Autodesk Fusion 360 part; units mm, degrees
(part 4 of 5)
  spline S1159 degree 3 poles (4.1337, -1.152) (3.9623, -1.0527) (3.8179, -1.0076) (3.8179, -1.0527) knots 0 0 0 0 1 1 1 1
  spline S1160 degree 3 poles (3.8179, -1.0527) (3.8179, -1.2062) (4.224, -1.5762) (4.3323, -1.5311) knots 0 0 0 0 1 1 1 1
  spline S1161 degree 3 poles (23.384, -1.3506) (23.5284, -1.2964) (24.1241, -0.5203) (24.1241, -0.3939) knots 0 0 0 0 1 1 1 1
  spline S1162 degree 3 poles (24.1241, -0.3939) (24.1241, -0.3398) (23.9797, -0.43) (23.8082, -0.6015) knots 0 0 0 0 1 1 1 1
  spline S1163 degree 3 poles (23.8082, -0.6015) (23.4562, -0.9444) (23.4021, -0.8813) (23.6728, -0.4481) knots 0 0 0 0 1 1 1 1
  spline S1164 degree 3 poles (23.6728, -0.4481) (23.9075, -0.06) (23.7721, -0.069) (23.5284, -0.4571) knots 0 0 0 0 1 1 1 1
  spline S1165 degree 3 poles (23.5284, -0.4571) (23.384, -0.6827) (23.1584, -1.4408) (23.2487, -1.4047) knots 0 0 0 0 1 1 1 1
  spline S1166 degree 3 poles (23.2487, -1.4047) (23.2577, -1.4047) (23.3209, -1.3776) (23.384, -1.3506) knots 0 0 0 0 1 1 1 1
  spline S1167 degree 3 poles (7.2203, -1.3506) (7.4188, -1.2784) (7.3557, -0.9625) (7.1571, -0.9625) knots 0 0 0 0 1 1 1 1
  spline S1168 degree 3 poles (7.1571, -0.9625) (7.0398, -0.9625) (6.9766, -1.0257) (6.9766, -1.134) knots 0 0 0 0 1 1 1 1
  spline S1169 degree 3 poles (6.9766, -1.134) (6.9766, -1.3325) (7.0578, -1.4047) (7.2203, -1.3506) knots 0 0 0 0 1 1 1 1
  spline S1170 degree 3 poles (22.4725, -1.1159) (22.8425, -0.9174) (23.4653, -0.2766) (23.1855, -0.3849) knots 0 0 0 0 1 1 1 1
  spline S1171 degree 3 poles (23.1855, -0.3849) (23.1043, -0.412) (23.0411, -0.3939) (23.0411, -0.3398) knots 0 0 0 0 1 1 1 1
  spline S1172 degree 3 poles (23.0411, -0.3398) (23.0411, -0.2856) (22.996, -0.2405) (22.9508, -0.2405) knots 0 0 0 0 1 1 1 1
  spline S1173 degree 3 poles (22.9508, -0.2405) (22.8967, -0.2405) (22.8696, -0.2676) (22.8786, -0.3127) knots 0 0 0 0 1 1 1 1
  spline S1174 degree 3 poles (22.8786, -0.3127) (22.8877, -0.3488) (22.8245, -0.5022) (22.7433, -0.6647) knots 0 0 0 0 1 1 1 1
  spline S1175 degree 3 poles (22.7433, -0.6647) (22.5898, -0.9535) (22.3462, -1.0888) (21.9852, -1.0979) knots 0 0 0 0 1 1 1 1
  spline S1176 degree 3 poles (21.9852, -1.0979) (21.8678, -1.0979) (21.7686, -1.143) (21.7595, -1.1881) knots 0 0 0 0 1 1 1 1
  spline S1177 degree 3 poles (21.7595, -1.1881) (21.7144, -1.3596) (22.0935, -1.3235) (22.4725, -1.1159) knots 0 0 0 0 1 1 1 1
  spline S1178 degree 3 poles (-3.6278, -1.2332) (-3.6007, -1.1881) (-3.6187, -1.143) (-3.6639, -1.143) knots 0 0 0 0 1 1 1 1
  spline S1179 degree 3 poles (-3.6639, -1.143) (-3.718, -1.143) (-3.7631, -1.1881) (-3.7631, -1.2332) knots 0 0 0 0 1 1 1 1
  spline S1180 degree 3 poles (-3.7631, -1.2332) (-3.7631, -1.2874) (-3.7451, -1.3235) (-3.727, -1.3235) knots 0 0 0 0 1 1 1 1
  spline S1181 degree 3 poles (-3.727, -1.3235) (-3.7, -1.3235) (-3.6548, -1.2874) (-3.6278, -1.2332) knots 0 0 0 0 1 1 1 1
  spline S1182 degree 3 poles (5.5326, -1.152) (5.5326, -1.0979) (5.307, -0.9083) (5.0362, -0.7278) knots 0 0 0 0 1 1 1 1
  spline S1183 degree 3 poles (5.0362, -0.7278) (4.6843, -0.4932) (4.5399, -0.3398) (4.5399, -0.1954) knots 0 0 0 0 1 1 1 1
  spline S1184 degree 3 poles (4.5399, -0.1954) (4.5399, -0.0871) (4.4406, 0.1476) (4.3233, 0.3281) knots 0 0 0 0 1 1 1 1
  spline S1185 degree 3 poles (4.3233, 0.3281) (4.1518, 0.5808) (4.1067, 0.7252) (4.1518, 0.9779) knots 0 0 0 0 1 1 1 1
  spline S1186 degree 3 poles (4.1518, 0.9779) (4.1879, 1.1945) (4.1698, 1.2938) (4.0886, 1.2938) knots 0 0 0 0 1 1 1 1
  spline S1187 degree 3 poles (4.0886, 1.2938) (4.0074, 1.2938) (3.9893, 1.393) (4.0254, 1.6277) knots 0 0 0 0 1 1 1 1
  spline S1188 degree 3 poles (4.0254, 1.6277) (4.0706, 1.9345) (4.0706, 1.9526) (3.9532, 1.8082) knots 0 0 0 0 1 1 1 1
  spline S1189 degree 3 poles (3.9532, 1.8082) (3.8359, 1.6457) (3.8269, 1.6548) (3.7998, 1.8533) knots 0 0 0 0 1 1 1 1
  spline S1190 degree 3 poles (3.7998, 1.8533) (3.7818, 1.9706) (3.8179, 2.2414) (3.881, 2.458) knots 0 0 0 0 1 1 1 1
  spline S1191 degree 3 poles (3.881, 2.458) (3.9713, 2.8009) (3.9713, 2.837) (3.863, 2.7287) knots 0 0 0 0 1 1 1 1
  spline S1192 degree 3 poles (3.863, 2.7287) (3.7908, 2.6565) (3.6735, 2.476) (3.5922, 2.3316) knots 0 0 0 0 1 1 1 1
  line L74 (3.5922, 2.3316) -> (3.4388, 2.0609)
  line L75 (3.4388, 2.0609) -> (3.4839, 2.3768)
  spline S1193 degree 3 poles (3.4839, 2.3768) (3.52, 2.6475) (3.502, 2.7017) (3.3666, 2.7107) knots 0 0 0 0 1 1 1 1
  spline S1194 degree 3 poles (3.3666, 2.7107) (3.2673, 2.7197) (3.1681, 2.6475) (3.141, 2.5482) knots 0 0 0 0 1 1 1 1
  spline S1195 degree 3 poles (3.141, 2.5482) (3.0688, 2.3316) (3.2764, 1.7721) (3.3666, 1.9255) knots 0 0 0 0 1 1 1 1
  spline S1196 degree 3 poles (3.3666, 1.9255) (3.3937, 1.9706) (3.4298, 1.7811) (3.4388, 1.5013) knots 0 0 0 0 1 1 1 1
  spline S1197 degree 3 poles (3.4388, 1.5013) (3.4478, 1.1494) (3.5291, 0.8335) (3.6825, 0.5357) knots 0 0 0 0 1 1 1 1
  spline S1198 degree 3 poles (3.6825, 0.5357) (3.8088, 0.292) (3.9081, 0.0122) (3.9081, -0.069) knots 0 0 0 0 1 1 1 1
  spline S1199 degree 3 poles (3.9081, -0.069) (3.9081, -0.1593) (3.9984, -0.2946) (4.1067, -0.3578) knots 0 0 0 0 1 1 1 1
  spline S1200 degree 3 poles (4.1067, -0.3578) (4.224, -0.43) (4.4947, -0.5925) (4.7204, -0.7278) knots 0 0 0 0 1 1 1 1
  spline S1201 degree 3 poles (4.7204, -0.7278) (4.946, -0.8542) (5.2167, -1.0257) (5.325, -1.1069) knots 0 0 0 0 1 1 1 1
  spline S1202 degree 3 poles (5.325, -1.1069) (5.4514, -1.1971) (5.5326, -1.2152) (5.5326, -1.152) knots 0 0 0 0 1 1 1 1
  spline S1203 degree 3 poles (1.0652, -1.0618) (1.1284, -0.9535) (0.7855, -0.8361) (0.6591, -0.9174) knots 0 0 0 0 1 1 1 1
  spline S1204 degree 3 poles (0.6591, -0.9174) (0.614, -0.9444) (0.5689, -1.0076) (0.5689, -1.0618) knots 0 0 0 0 1 1 1 1
  spline S1205 degree 3 poles (0.5689, -1.0618) (0.5689, -1.1701) (0.993, -1.1701) (1.0652, -1.0618) knots 0 0 0 0 1 1 1 1
  spline S1206 degree 3 poles (-3.2036, -0.8993) (-3.0141, -0.8271) (-2.8606, -0.7098) (-2.8606, -0.6466) knots 0 0 0 0 1 1 1 1
  spline S1207 degree 3 poles (-2.8606, -0.6466) (-2.8606, -0.5834) (-2.7162, -0.439) (-2.5448, -0.3307) knots 0 0 0 0 1 1 1 1
  spline S1208 degree 3 poles (-2.5448, -0.3307) (-2.3733, -0.2224) (-2.2469, -0.0961) (-2.283, -0.051) knots 0 0 0 0 1 1 1 1
  spline S1209 degree 3 poles (-2.283, -0.051) (-2.3462, 0.0573) (-2.5899, 0.0573) (-2.5899, -0.051) knots 0 0 0 0 1 1 1 1
  spline S1210 degree 3 poles (-2.5899, -0.051) (-2.5899, -0.1051) (-2.7614, -0.1502) (-2.978, -0.1683) knots 0 0 0 0 1 1 1 1
  spline S1211 degree 3 poles (-2.978, -0.1683) (-3.2938, -0.1863) (-3.366, -0.2315) (-3.3841, -0.4029) knots 0 0 0 0 1 1 1 1
  spline S1212 degree 3 poles (-3.3841, -0.4029) (-3.4112, -0.5564) (-3.4743, -0.6015) (-3.6729, -0.6015) knots 0 0 0 0 1 1 1 1
  spline S1213 degree 3 poles (-3.6729, -0.6015) (-3.9978, -0.6015) (-4.079, -0.7188) (-3.8895, -0.9083) knots 0 0 0 0 1 1 1 1
  spline S1214 degree 3 poles (-3.8895, -0.9083) (-3.718, -1.0798) (-3.6368, -1.0798) (-3.2036, -0.8993) knots 0 0 0 0 1 1 1 1
  spline S1215 degree 3 poles (24.449, -0.6737) (24.7288, -0.3578) (24.9544, 0.0393) (24.8912, 0.1025) knots 0 0 0 0 1 1 1 1
  spline S1216 degree 3 poles (24.8912, 0.1025) (24.828, 0.1747) (24.1331, -0.6015) (24.1241, -0.7639) knots 0 0 0 0 1 1 1 1
  spline S1217 degree 3 poles (24.1241, -0.7639) (24.1241, -0.9354) (24.2504, -0.8903) (24.449, -0.6737) knots 0 0 0 0 1 1 1 1
  spline S1218 degree 3 poles (22.4093, -0.6917) (22.5086, -0.6195) (22.4725, -0.6105) (22.274, -0.6556) knots 0 0 0 0 1 1 1 1
  spline S1219 degree 3 poles (22.274, -0.6556) (21.94, -0.7278) (21.8678, -0.782) (22.1025, -0.782) knots 0 0 0 0 1 1 1 1
  spline S1220 degree 3 poles (22.1025, -0.782) (22.1927, -0.782) (22.3371, -0.7369) (22.4093, -0.6917) knots 0 0 0 0 1 1 1 1
  spline S1221 degree 3 poles (-1.4166, -0.5473) (-1.2, -0.421) (-0.8932, -0.3037) (-0.7398, -0.2856) knots 0 0 0 0 1 1 1 1
  spline S1222 degree 3 poles (-0.7398, -0.2856) (0.1447, -0.1683) (1.0652, 0.1025) (1.6428, 0.4274) knots 0 0 0 0 1 1 1 1
  line L76 (1.6428, 0.4274) -> (1.8594, 0.5447)
  line L77 (1.8594, 0.5447) -> (1.6609, 0.653)
  spline S1223 degree 3 poles (1.6609, 0.653) (1.5526, 0.7162) (1.345, 0.7432) (1.2006, 0.7071) knots 0 0 0 0 1 1 1 1
  spline S1224 degree 3 poles (1.2006, 0.7071) (0.8757, 0.6349) (0.7674, 0.7974) (0.984, 1.032) knots 0 0 0 0 1 1 1 1
  spline S1225 degree 3 poles (0.984, 1.032) (1.0833, 1.1403) (1.1013, 1.2035) (1.0291, 1.2035) knots 0 0 0 0 1 1 1 1
  spline S1226 degree 3 poles (1.0291, 1.2035) (0.8938, 1.2035) (0.6591, 0.9779) (0.6591, 0.8515) knots 0 0 0 0 1 1 1 1
  spline S1227 degree 3 poles (0.6591, 0.8515) (0.6591, 0.7613) (0.1627, 0.4815) (0.0003, 0.4815) knots 0 0 0 0 1 1 1 1
  spline S1228 degree 3 poles (0.0003, 0.4815) (-0.0448, 0.4815) (-0.2163, 0.3371) (-0.3697, 0.1566) knots 0 0 0 0 1 1 1 1
  spline S1229 degree 3 poles (-0.3697, 0.1566) (-0.5954, -0.1051) (-0.7217, -0.1683) (-1.0105, -0.1863) knots 0 0 0 0 1 1 1 1
  spline S1230 degree 3 poles (-1.0105, -0.1863) (-1.2722, -0.2044) (-1.4527, -0.2856) (-1.6784, -0.4932) knots 0 0 0 0 1 1 1 1
  spline S1231 degree 3 poles (-1.6784, -0.4932) (-2.0394, -0.8452) (-1.9581, -0.8542) (-1.4166, -0.5473) knots 0 0 0 0 1 1 1 1
  spline S1232 degree 3 poles (25.3876, -0.2405) (25.3154, 0.0212) (25.3244, 0.0303) (25.541, -0.0239) knots 0 0 0 0 1 1 1 1
  spline S1233 degree 3 poles (25.541, -0.0239) (25.7035, -0.069) (25.7576, -0.051) (25.7125, 0.0212) knots 0 0 0 0 1 1 1 1
  spline S1234 degree 3 poles (25.7125, 0.0212) (25.6403, 0.1295) (25.1168, 0.1566) (25.1168, 0.0483) knots 0 0 0 0 1 1 1 1
  spline S1235 degree 3 poles (25.1168, 0.0483) (25.1168, -0.078) (25.3425, -0.5112) (25.4056, -0.5112) knots 0 0 0 0 1 1 1 1
  spline S1236 degree 3 poles (25.4056, -0.5112) (25.4417, -0.5112) (25.4327, -0.3849) (25.3876, -0.2405) knots 0 0 0 0 1 1 1 1
  spline S1237 degree 3 poles (3.3937, -0.2315) (3.3395, 0.0393) (2.9334, 0.5718) (2.789, 0.5718) knots 0 0 0 0 1 1 1 1
  spline S1238 degree 3 poles (2.789, 0.5718) (2.7078, 0.5718) (2.7258, 0.1566) (2.8251, -0.1051) knots 0 0 0 0 1 1 1 1
  spline S1239 degree 3 poles (2.8251, -0.1051) (2.8793, -0.2405) (2.9605, -0.3127) (3.0146, -0.2856) knots 0 0 0 0 1 1 1 1
  spline S1240 degree 3 poles (3.0146, -0.2856) (3.0598, -0.2495) (3.1861, -0.2946) (3.2854, -0.3849) knots 0 0 0 0 1 1 1 1
  spline S1241 degree 3 poles (3.2854, -0.3849) (3.4569, -0.5383) (3.4569, -0.5293) (3.3937, -0.2315) knots 0 0 0 0 1 1 1 1
  spline S1242 degree 3 poles (5.5687, 0.0573) (5.6138, 0.31) (5.5958, 0.4454) (5.5146, 0.4905) knots 0 0 0 0 1 1 1 1
  spline S1243 degree 3 poles (5.5146, 0.4905) (5.4514, 0.5357) (5.4153, 0.6981) (5.4333, 0.8876) knots 0 0 0 0 1 1 1 1
  line L78 (5.4333, 0.8876) -> (5.4604, 1.2216)
  line L79 (5.4604, 1.2216) -> (5.2619, 1.023)
  spline S1244 degree 3 poles (5.2619, 1.023) (5.0994, 0.8606) (5.0814, 0.7884) (5.1536, 0.6169) knots 0 0 0 0 1 1 1 1
  spline S1245 degree 3 poles (5.1536, 0.6169) (5.2077, 0.4996) (5.2258, 0.2649) (5.1987, 0.0934) knots 0 0 0 0 1 1 1 1
  spline S1246 degree 3 poles (5.1987, 0.0934) (5.1626, -0.1593) (5.1806, -0.2224) (5.3341, -0.2585) knots 0 0 0 0 1 1 1 1
  spline S1247 degree 3 poles (5.3341, -0.2585) (5.4875, -0.3037) (5.5236, -0.2495) (5.5687, 0.0573) knots 0 0 0 0 1 1 1 1
  spline S1248 degree 3 poles (1.5165, -0.2405) (1.5436, -0.1954) (1.5345, -0.1502) (1.4804, -0.1502) knots 0 0 0 0 1 1 1 1
  spline S1249 degree 3 poles (1.4804, -0.1502) (1.4353, -0.1502) (1.3631, -0.1954) (1.336, -0.2405) knots 0 0 0 0 1 1 1 1
  spline S1250 degree 3 poles (1.336, -0.2405) (1.3089, -0.2946) (1.3179, -0.3307) (1.3721, -0.3307) knots 0 0 0 0 1 1 1 1
  spline S1251 degree 3 poles (1.3721, -0.3307) (1.4172, -0.3307) (1.4894, -0.2946) (1.5165, -0.2405) knots 0 0 0 0 1 1 1 1
  spline S1252 degree 3 poles (24.3768, -0.0871) (24.44, -0.069) (24.5302, 0.0393) (24.5844, 0.1386) knots 0 0 0 0 1 1 1 1
  spline S1253 degree 3 poles (24.5844, 0.1386) (24.6836, 0.3191) (24.6746, 0.3191) (24.4039, 0.1295) knots 0 0 0 0 1 1 1 1
  spline S1254 degree 3 poles (24.4039, 0.1295) (24.0519, -0.1232) (24.0338, -0.2224) (24.3768, -0.0871) knots 0 0 0 0 1 1 1 1
  spline S1255 degree 3 poles (8.4748, -0.051) (8.5018, 0.0032) (8.4838, 0.0934) (8.4296, 0.1476) knots 0 0 0 0 1 1 1 1
  spline S1256 degree 3 poles (8.4296, 0.1476) (8.3574, 0.2198) (8.3304, 0.1927) (8.3304, 0.0483) knots 0 0 0 0 1 1 1 1
  spline S1257 degree 3 poles (8.3304, 0.0483) (8.3304, -0.1683) (8.3755, -0.2044) (8.4748, -0.051) knots 0 0 0 0 1 1 1 1
  spline S1258 degree 3 poles (6.1644, 0.31) (6.1644, 0.5176) (5.9297, 0.7974) (5.8575, 0.6801) knots 0 0 0 0 1 1 1 1
  spline S1259 degree 3 poles (5.8575, 0.6801) (5.7853, 0.5537) (5.9026, 0.2288) (6.038, 0.1747) knots 0 0 0 0 1 1 1 1
  spline S1260 degree 3 poles (6.038, 0.1747) (6.1192, 0.1386) (6.1644, 0.1927) (6.1644, 0.31) knots 0 0 0 0 1 1 1 1
  spline S1261 degree 3 poles (-1.7325, 0.4815) (-1.6964, 0.5357) (-1.7776, 0.5718) (-1.904, 0.5718) knots 0 0 0 0 1 1 1 1
  spline S1262 degree 3 poles (-1.904, 0.5718) (-2.0303, 0.5718) (-2.1386, 0.5266) (-2.1386, 0.4815) knots 0 0 0 0 1 1 1 1
  spline S1263 degree 3 poles (-2.1386, 0.4815) (-2.1386, 0.4274) (-2.0574, 0.3913) (-1.9672, 0.3913) knots 0 0 0 0 1 1 1 1
  spline S1264 degree 3 poles (-1.9672, 0.3913) (-1.8679, 0.3913) (-1.7596, 0.4274) (-1.7325, 0.4815) knots 0 0 0 0 1 1 1 1
  spline S1265 degree 3 poles (7.7889, 0.5718) (7.7889, 0.6169) (7.7437, 0.662) (7.6986, 0.662) knots 0 0 0 0 1 1 1 1
  spline S1266 degree 3 poles (7.6986, 0.662) (7.6445, 0.662) (7.6084, 0.6169) (7.6084, 0.5718) knots 0 0 0 0 1 1 1 1
  spline S1267 degree 3 poles (7.6084, 0.5718) (7.6084, 0.5176) (7.6445, 0.4815) (7.6986, 0.4815) knots 0 0 0 0 1 1 1 1
  spline S1268 degree 3 poles (7.6986, 0.4815) (7.7437, 0.4815) (7.7889, 0.5176) (7.7889, 0.5718) knots 0 0 0 0 1 1 1 1
  spline S1269 degree 3 poles (25.9291, 0.7703) (25.9291, 0.8515) (25.884, 0.9508) (25.8388, 0.9779) knots 0 0 0 0 1 1 1 1
  spline S1270 degree 3 poles (25.8388, 0.9779) (25.7847, 1.005) (25.7486, 1.1855) (25.7486, 1.366) knots 0 0 0 0 1 1 1 1
  spline S1271 degree 3 poles (25.7486, 1.366) (25.7486, 1.7631) (25.6222, 2.0158) (25.541, 1.8082) knots 0 0 0 0 1 1 1 1
  spline S1272 degree 3 poles (25.541, 1.8082) (25.5139, 1.7179) (25.4237, 1.6909) (25.3154, 1.7179) knots 0 0 0 0 1 1 1 1
  spline S1273 degree 3 poles (25.3154, 1.7179) (25.2161, 1.736) (25.1078, 1.7179) (25.0717, 1.6548) knots 0 0 0 0 1 1 1 1
  spline S1274 degree 3 poles (25.0717, 1.6548) (25.0356, 1.5916) (25.0807, 1.5284) (25.1981, 1.5013) knots 0 0 0 0 1 1 1 1
  spline S1275 degree 3 poles (25.1981, 1.5013) (25.3154, 1.4743) (25.4147, 1.3479) (25.4598, 1.1674) knots 0 0 0 0 1 1 1 1
  spline S1276 degree 3 poles (25.4598, 1.1674) (25.5049, 1.014) (25.5861, 0.8876) (25.6493, 0.8876) knots 0 0 0 0 1 1 1 1
  spline S1277 degree 3 poles (25.6493, 0.8876) (25.7035, 0.8876) (25.7937, 0.8245) (25.8388, 0.7523) knots 0 0 0 0 1 1 1 1
  spline S1278 degree 3 poles (25.8388, 0.7523) (25.911, 0.6349) (25.9291, 0.6349) (25.9291, 0.7703) knots 0 0 0 0 1 1 1 1
  spline S1279 degree 3 poles (25.3244, 0.7252) (25.3695, 0.8064) (25.2342, 1.2035) (25.162, 1.2035) knots 0 0 0 0 1 1 1 1
  spline S1280 degree 3 poles (25.162, 1.2035) (25.1349, 1.2035) (25.1168, 1.0772) (25.1168, 0.9328) knots 0 0 0 0 1 1 1 1
  spline S1281 degree 3 poles (25.1168, 0.9328) (25.1168, 0.6801) (25.2342, 0.5718) (25.3244, 0.7252) knots 0 0 0 0 1 1 1 1
  spline S1282 degree 3 poles (24.9363, 0.7974) (24.9363, 0.8696) (24.9002, 0.9328) (24.8461, 0.9328) knots 0 0 0 0 1 1 1 1
  spline S1283 degree 3 poles (24.8461, 0.9328) (24.801, 0.9328) (24.7829, 0.8696) (24.81, 0.7974) knots 0 0 0 0 1 1 1 1
  spline S1284 degree 3 poles (24.81, 0.7974) (24.8461, 0.7252) (24.8822, 0.662) (24.9002, 0.662) knots 0 0 0 0 1 1 1 1
  spline S1285 degree 3 poles (24.9002, 0.662) (24.9183, 0.662) (24.9363, 0.7252) (24.9363, 0.7974) knots 0 0 0 0 1 1 1 1
  spline S1286 degree 3 poles (-4.0068, 0.9057) (-4.088, 1.1494) (-4.2234, 1.2938) (-4.3588, 1.2938) knots 0 0 0 0 1 1 1 1
  spline S1287 degree 3 poles (-4.3588, 1.2938) (-4.5483, 1.2938) (-4.5122, 1.1223) (-4.2866, 0.9237) knots 0 0 0 0 1 1 1 1
  spline S1288 degree 3 poles (-4.2866, 0.9237) (-4.0249, 0.7162) (-3.9346, 0.7071) (-4.0068, 0.9057) knots 0 0 0 0 1 1 1 1
  spline S1289 degree 3 poles (2.8432, 1.1494) (2.9154, 1.5284) (2.5273, 1.736) (2.419, 1.384) knots 0 0 0 0 1 1 1 1
  spline S1290 degree 3 poles (2.419, 1.384) (2.3558, 1.1764) (2.437, 0.9959) (2.5634, 1.0681) knots 0 0 0 0 1 1 1 1
  spline S1291 degree 3 poles (2.5634, 1.0681) (2.6085, 1.1042) (2.6446, 1.0772) (2.6446, 1.032) knots 0 0 0 0 1 1 1 1
  spline S1292 degree 3 poles (2.6446, 1.032) (2.6446, 0.8425) (2.8071, 0.9418) (2.8432, 1.1494) knots 0 0 0 0 1 1 1 1
  spline S1293 degree 3 poles (-3.2397, 1.1313) (-3.3029, 1.2486) (-3.4202, 1.384) (-3.4924, 1.4472) knots 0 0 0 0 1 1 1 1
  spline S1294 degree 3 poles (-3.4924, 1.4472) (-3.6097, 1.5465) (-3.6007, 1.5555) (-3.4292, 1.5645) knots 0 0 0 0 1 1 1 1
  spline S1295 degree 3 poles (-3.4292, 1.5645) (-3.0592, 1.5645) (-3.2126, 1.7992) (-3.7902, 2.106) knots 0 0 0 0 1 1 1 1
  spline S1296 degree 3 poles (-3.7902, 2.106) (-3.9436, 2.1872) (-4.1332, 2.3677) (-4.1963, 2.5031) knots 0 0 0 0 1 1 1 1
  spline S1297 degree 3 poles (-4.1963, 2.5031) (-4.2595, 2.6295) (-4.3588, 2.7378) (-4.4039, 2.7378) knots 0 0 0 0 1 1 1 1
  spline S1298 degree 3 poles (-4.4039, 2.7378) (-4.4581, 2.7378) (-4.4761, 2.7017) (-4.449, 2.6565) knots 0 0 0 0 1 1 1 1
  spline S1299 degree 3 poles (-4.449, 2.6565) (-4.4129, 2.6114) (-4.44, 2.5573) (-4.4942, 2.5392) knots 0 0 0 0 1 1 1 1
  spline S1300 degree 3 poles (-4.4942, 2.5392) (-4.6386, 2.4941) (-3.8805, 1.4111) (-3.5736, 1.2306) knots 0 0 0 0 1 1 1 1
  spline S1301 degree 3 poles (-3.5736, 1.2306) (-3.4292, 1.1403) (-3.3119, 1.0411) (-3.3119, 1.005) knots 0 0 0 0 1 1 1 1
  spline S1302 degree 3 poles (-3.3119, 1.005) (-3.3119, 0.9689) (-3.2668, 0.9328) (-3.2216, 0.9328) knots 0 0 0 0 1 1 1 1
  spline S1303 degree 3 poles (-3.2216, 0.9328) (-3.1675, 0.9328) (-3.1765, 1.014) (-3.2397, 1.1313) knots 0 0 0 0 1 1 1 1
  spline S1304 degree 3 poles (7.9513, 1.5284) (7.9333, 1.8804) (7.8881, 1.9797) (7.7528, 1.9977) knots 0 0 0 0 1 1 1 1
  spline S1305 degree 3 poles (7.7528, 1.9977) (7.6174, 2.0248) (7.5993, 1.9977) (7.6535, 1.8714) knots 0 0 0 0 1 1 1 1
  spline S1306 degree 3 poles (7.6535, 1.8714) (7.6896, 1.7721) (7.7437, 1.5916) (7.7708, 1.4472) knots 0 0 0 0 1 1 1 1
  spline S1307 degree 3 poles (7.7708, 1.4472) (7.843, 1.014) (7.9784, 1.0681) (7.9513, 1.5284) knots 0 0 0 0 1 1 1 1
  spline S1308 degree 3 poles (5.3521, 1.6096) (5.4333, 1.754) (5.5507, 1.8804) (5.6229, 1.8804) knots 0 0 0 0 1 1 1 1
  spline S1309 degree 3 poles (5.6229, 1.8804) (5.8304, 1.8894) (5.9839, 2.0067) (5.9839, 2.1692) knots 0 0 0 0 1 1 1 1
  spline S1310 degree 3 poles (5.9839, 2.1692) (5.9839, 2.2504) (6.0561, 2.3948) (6.1373, 2.4941) knots 0 0 0 0 1 1 1 1
  spline S1311 degree 3 poles (6.1373, 2.4941) (6.2907, 2.6656) (6.2907, 2.6746) (6.0922, 2.6295) knots 0 0 0 0 1 1 1 1
  spline S1312 degree 3 poles (6.0922, 2.6295) (5.8665, 2.5663) (5.8575, 2.5843) (5.9839, 2.837) knots 0 0 0 0 1 1 1 1
  spline S1313 degree 3 poles (5.9839, 2.837) (6.1373, 3.1168) (5.9568, 3.0356) (5.686, 2.6926) knots 0 0 0 0 1 1 1 1
  spline S1314 degree 3 poles (5.686, 2.6926) (5.3702, 2.2955) (5.1536, 1.7901) (5.1897, 1.5284) knots 0 0 0 0 1 1 1 1
  spline S1315 degree 3 poles (5.1897, 1.5284) (5.2167, 1.3569) (5.2348, 1.366) (5.3521, 1.6096) knots 0 0 0 0 1 1 1 1
  spline S1316 degree 3 poles (-0.8751, 1.6728) (-0.3697, 1.8082) (-0.3697, 1.9075) (-0.8661, 1.9345) knots 0 0 0 0 1 1 1 1
  spline S1317 degree 3 poles (-0.8661, 1.9345) (-1.2091, 1.9616) (-1.3174, 1.9436) (-1.2813, 1.8533) knots 0 0 0 0 1 1 1 1
  spline S1318 degree 3 poles (-1.2813, 1.8533) (-1.2632, 1.7992) (-1.2813, 1.745) (-1.3264, 1.745) knots 0 0 0 0 1 1 1 1
  spline S1319 degree 3 poles (-1.3264, 1.745) (-1.3805, 1.745) (-1.4166, 1.6999) (-1.4166, 1.6548) knots 0 0 0 0 1 1 1 1
  spline S1320 degree 3 poles (-1.4166, 1.6548) (-1.4166, 1.5465) (-1.2993, 1.5465) (-0.8751, 1.6728) knots 0 0 0 0 1 1 1 1
  spline S1321 degree 3 poles (-2.7253, 1.8353) (-2.7523, 1.8804) (-2.8426, 1.9255) (-2.9148, 1.9255) knots 0 0 0 0 1 1 1 1
  spline S1322 degree 3 poles (-2.9148, 1.9255) (-2.987, 1.9255) (-3.0231, 1.8804) (-2.996, 1.8353) knots 0 0 0 0 1 1 1 1
  spline S1323 degree 3 poles (-2.996, 1.8353) (-2.9689, 1.7811) (-2.8787, 1.745) (-2.8065, 1.745) knots 0 0 0 0 1 1 1 1
  spline S1324 degree 3 poles (-2.8065, 1.745) (-2.7343, 1.745) (-2.6982, 1.7811) (-2.7253, 1.8353) knots 0 0 0 0 1 1 1 1
  spline S1325 degree 3 poles (4.6662, 2.2143) (4.8648, 2.4851) (4.8467, 2.5573) (4.603, 2.5573) knots 0 0 0 0 1 1 1 1
  spline S1326 degree 3 poles (4.603, 2.5573) (4.4406, 2.5573) (4.4045, 2.5121) (4.4045, 2.3316) knots 0 0 0 0 1 1 1 1
  spline S1327 degree 3 poles (4.4045, 2.3316) (4.4225, 2.0067) (4.5038, 1.9706) (4.6662, 2.2143) knots 0 0 0 0 1 1 1 1
  spline S1328 degree 3 poles (-1.4166, 2.467) (-1.4166, 2.5121) (-1.4798, 2.5573) (-1.552, 2.5573) knots 0 0 0 0 1 1 1 1
  spline S1329 degree 3 poles (-1.552, 2.5573) (-1.6242, 2.5573) (-1.6874, 2.5121) (-1.6874, 2.467) knots 0 0 0 0 1 1 1 1
  spline S1330 degree 3 poles (-1.6874, 2.467) (-1.6874, 2.4129) (-1.6242, 2.3768) (-1.552, 2.3768) knots 0 0 0 0 1 1 1 1
  spline S1331 degree 3 poles (-1.552, 2.3768) (-1.4798, 2.3768) (-1.4166, 2.4129) (-1.4166, 2.467) knots 0 0 0 0 1 1 1 1
  spline S1332 degree 3 poles (8.1318, 2.5753) (8.2762, 2.7197) (8.2672, 2.9183) (8.1138, 2.9183) knots 0 0 0 0 1 1 1 1
  spline S1333 degree 3 poles (8.1138, 2.9183) (7.9333, 2.9183) (7.852, 2.7648) (7.9423, 2.6024) knots 0 0 0 0 1 1 1 1
  spline S1334 degree 3 poles (7.9423, 2.6024) (8.0055, 2.4941) (8.0506, 2.4941) (8.1318, 2.5753) knots 0 0 0 0 1 1 1 1
  spline S1335 degree 3 poles (2.2385, 2.9183) (2.2656, 2.9634) (2.2114, 3.0085) (2.1121, 3.0085) knots 0 0 0 0 1 1 1 1
  spline S1336 degree 3 poles (2.1121, 3.0085) (2.0038, 3.0085) (1.9226, 2.9634) (1.9226, 2.9183) knots 0 0 0 0 1 1 1 1
  spline S1337 degree 3 poles (1.9226, 2.9183) (1.9226, 2.8641) (1.9768, 2.828) (2.049, 2.828) knots 0 0 0 0 1 1 1 1
  spline S1338 degree 3 poles (2.049, 2.828) (2.1212, 2.828) (2.2114, 2.8641) (2.2385, 2.9183) knots 0 0 0 0 1 1 1 1
  spline S1339 degree 3 poles (-12.2466, 2.9995) (-12.2466, 3.1078) (-12.3008, 3.189) (-12.391, 3.189) knots 0 0 0 0 1 1 1 1
  spline S1340 degree 3 poles (-12.391, 3.189) (-12.4723, 3.189) (-12.5174, 3.1258) (-12.4993, 3.0356) knots 0 0 0 0 1 1 1 1
  spline S1341 degree 3 poles (-12.4993, 3.0356) (-12.4542, 2.81) (-12.2466, 2.7829) (-12.2466, 2.9995) knots 0 0 0 0 1 1 1 1
  spline S1342 degree 3 poles (-6.1999, -2.6141) (-5.7035, -2.5419) (-5.5862, -2.4877) (-5.532, -2.3523) knots 0 0 0 0 1 1 1 1
  spline S1343 degree 3 poles (-5.532, -2.3523) (-5.4237, -2.0816) (-5.5681, -1.874) (-5.893, -1.8108) knots 0 0 0 0 1 1 1 1
  line L80 (-5.893, -1.8108) -> (-6.1999, -1.7567)
  line L81 (-6.1999, -1.7567) -> (-5.9743, -1.5401)
  spline S1344 degree 3 poles (-5.9743, -1.5401) (-5.6042, -1.1971) (-5.7486, -0.6015) (-6.1999, -0.6015) knots 0 0 0 0 1 1 1 1
  spline S1345 degree 3 poles (-6.1999, -0.6015) (-6.4165, -0.6015) (-7.4724, -1.143) (-7.7612, -1.3957) knots 0 0 0 0 1 1 1 1
  spline S1346 degree 3 poles (-7.7612, -1.3957) (-7.9959, -1.6033) (-7.9507, -1.856) (-7.6078, -2.1718) knots 0 0 0 0 1 1 1 1
  spline S1347 degree 3 poles (-7.6078, -2.1718) (-7.3461, -2.4245) (-6.7324, -2.6953) (-6.5067, -2.6682) knots 0 0 0 0 1 1 1 1
  spline S1348 degree 3 poles (-6.5067, -2.6682) (-6.4616, -2.6592) (-6.3262, -2.6411) (-6.1999, -2.6141) knots 0 0 0 0 1 1 1 1
  spline S1349 degree 3 poles (-7.6439, -1.9733) (-7.6439, -1.7928) (-6.3714, -1.0527) (-6.0645, -1.0527) knots 0 0 0 0 1 1 1 1
  spline S1350 degree 3 poles (-6.0645, -1.0527) (-5.884, -1.0527) (-5.893, -1.2603) (-6.0916, -1.4408) knots 0 0 0 0 1 1 1 1
  spline S1351 degree 3 poles (-6.0916, -1.4408) (-6.4706, -1.7838) (-7.6439, -2.1899) (-7.6439, -1.9733) knots 0 0 0 0 1 1 1 1
  spline S1352 degree 3 poles (-6.1999, -1.4137) (-6.1277, -1.3686) (-6.1006, -1.3054) (-6.1367, -1.2693) knots 0 0 0 0 1 1 1 1
  spline S1353 degree 3 poles (-6.1367, -1.2693) (-6.1728, -1.2332) (-6.254, -1.2513) (-6.3082, -1.3054) knots 0 0 0 0 1 1 1 1
  spline S1354 degree 3 poles (-6.3082, -1.3054) (-6.4436, -1.4408) (-6.3714, -1.522) (-6.1999, -1.4137) knots 0 0 0 0 1 1 1 1
  spline S1355 degree 3 poles (-11.0463, -2.3975) (-11.0824, -2.2801) (-11.1185, -2.235) (-11.1456, -2.3072) knots 0 0 0 0 1 1 1 1
  spline S1356 degree 3 poles (-11.1456, -2.3072) (-11.1636, -2.3704) (-11.1366, -2.4697) (-11.0914, -2.5148) knots 0 0 0 0 1 1 1 1
  spline S1357 degree 3 poles (-11.0914, -2.5148) (-11.0192, -2.587) (-11.0102, -2.5509) (-11.0463, -2.3975) knots 0 0 0 0 1 1 1 1
  spline S1358 degree 3 poles (-10.4597, -2.226) (-10.3875, -2.1087) (-10.4146, -1.9823) (-10.586, -1.6935) knots 0 0 0 0 1 1 1 1
  spline S1359 degree 3 poles (-10.586, -1.6935) (-10.8207, -1.3145) (-10.9831, -1.2152) (-10.9831, -1.4589) knots 0 0 0 0 1 1 1 1
  spline S1360 degree 3 poles (-10.9831, -1.4589) (-10.9831, -1.5311) (-11.0283, -1.5942) (-11.0734, -1.5942) knots 0 0 0 0 1 1 1 1
  spline S1361 degree 3 poles (-11.0734, -1.5942) (-11.2449, -1.5942) (-11.1636, -1.7657) (-10.8568, -2.0726) knots 0 0 0 0 1 1 1 1
  spline S1362 degree 3 poles (-10.8568, -2.0726) (-10.586, -2.3433) (-10.5499, -2.3614) (-10.4597, -2.226) knots 0 0 0 0 1 1 1 1
  spline S1363 degree 3 poles (-9.6835, -0.9805) (-9.6655, -0.9444) (-9.6835, -0.7188) (-9.7287, -0.4932) knots 0 0 0 0 1 1 1 1
  spline S1364 degree 3 poles (-9.7287, -0.4932) (-9.8099, -0.1322) (-9.7918, -0.0058) (-9.6384, 0.3552) knots 0 0 0 0 1 1 1 1
  spline S1365 degree 3 poles (-9.6384, 0.3552) (-9.5301, 0.5808) (-9.4489, 0.8425) (-9.4489, 0.9147) knots 0 0 0 0 1 1 1 1
  spline S1366 degree 3 poles (-9.4489, 0.9147) (-9.4489, 0.9959) (-9.3406, 1.1674) (-9.2052, 1.3118) knots 0 0 0 0 1 1 1 1
  spline S1367 degree 3 poles (-9.2052, 1.3118) (-9.0789, 1.4472) (-8.9976, 1.5916) (-9.0337, 1.6277) knots 0 0 0 0 1 1 1 1
  spline S1368 degree 3 poles (-9.0337, 1.6277) (-9.0698, 1.6638) (-9.2413, 1.5374) (-9.4038, 1.3389) knots 0 0 0 0 1 1 1 1
  spline S1369 degree 3 poles (-9.4038, 1.3389) (-9.6565, 1.0501) (-9.7287, 1.005) (-9.8009, 1.1042) knots 0 0 0 0 1 1 1 1
  spline S1370 degree 3 poles (-9.8009, 1.1042) (-9.8731, 1.2125) (-9.9092, 1.2125) (-10.0265, 1.1223) knots 0 0 0 0 1 1 1 1
  spline S1371 degree 3 poles (-10.0265, 1.1223) (-10.1889, 0.9869) (-10.216, 0.7884) (-10.0897, 0.7342) knots 0 0 0 0 1 1 1 1
  spline S1372 degree 3 poles (-10.0897, 0.7342) (-10.0445, 0.7162) (-10.0445, 0.4905) (-10.0987, 0.1837) knots 0 0 0 0 1 1 1 1
  spline S1373 degree 3 poles (-10.0987, 0.1837) (-10.1799, -0.2676) (-10.1709, -0.4029) (-10.0355, -0.7008) knots 0 0 0 0 1 1 1 1
  spline S1374 degree 3 poles (-10.0355, -0.7008) (-9.8731, -1.0437) (-9.7738, -1.1249) (-9.6835, -0.9805) knots 0 0 0 0 1 1 1 1
  spline S1375 degree 3 poles (-10.7485, -0.773) (-10.7214, -0.7188) (-10.7304, -0.6376) (-10.7756, -0.5925) knots 0 0 0 0 1 1 1 1
  spline S1376 degree 3 poles (-10.7756, -0.5925) (-10.8839, -0.4842) (-10.5319, 0.7884) (-10.225, 1.384) knots 0 0 0 0 1 1 1 1
  spline S1377 degree 3 poles (-10.225, 1.384) (-9.9904, 1.8353) (-9.8279, 2.3948) (-9.9723, 2.2414) knots 0 0 0 0 1 1 1 1
  spline S1378 degree 3 poles (-9.9723, 2.2414) (-10.568, 1.6277) (-10.8026, 1.2577) (-10.8026, 0.9598) knots 0 0 0 0 1 1 1 1
  spline S1379 degree 3 poles (-10.8026, 0.9598) (-10.8026, 0.7793) (-10.8568, 0.5898) (-10.929, 0.5357) knots 0 0 0 0 1 1 1 1
  spline S1380 degree 3 poles (-10.929, 0.5357) (-11.0734, 0.4183) (-11.2088, -0.1863) (-11.0734, -0.1051) knots 0 0 0 0 1 1 1 1
  spline S1381 degree 3 poles (-11.0734, -0.1051) (-11.0192, -0.069) (-10.9831, -0.2134) (-10.9831, -0.4571) knots 0 0 0 0 1 1 1 1
  spline S1382 degree 3 poles (-10.9831, -0.4571) (-10.9831, -0.8542) (-10.8839, -0.9896) (-10.7485, -0.773) knots 0 0 0 0 1 1 1 1
  spline S1383 degree 3 poles (-8.411, -0.3307) (-8.3839, -0.2856) (-8.402, -0.2405) (-8.4471, -0.2405) knots 0 0 0 0 1 1 1 1
  spline S1384 degree 3 poles (-8.4471, -0.2405) (-8.5013, -0.2405) (-8.5464, -0.2856) (-8.5464, -0.3307) knots 0 0 0 0 1 1 1 1
  spline S1385 degree 3 poles (-8.5464, -0.3307) (-8.5464, -0.3849) (-8.5283, -0.421) (-8.5103, -0.421) knots 0 0 0 0 1 1 1 1
  spline S1386 degree 3 poles (-8.5103, -0.421) (-8.4832, -0.421) (-8.4381, -0.3849) (-8.411, -0.3307) knots 0 0 0 0 1 1 1 1
  spline S1387 degree 3 poles (-7.7341, -0.1502) (-7.6258, -0.078) (-7.6349, -0.06) (-7.7973, -0.06) knots 0 0 0 0 1 1 1 1
  spline S1388 degree 3 poles (-7.7973, -0.06) (-7.9056, -0.06) (-8.0229, -0.1051) (-8.05, -0.1502) knots 0 0 0 0 1 1 1 1
  spline S1389 degree 3 poles (-8.05, -0.1502) (-8.1222, -0.2676) (-7.9146, -0.2676) (-7.7341, -0.1502) knots 0 0 0 0 1 1 1 1
  spline S1390 degree 3 poles (-7.0753, 0.1295) (-6.8948, 0.2288) (-6.5519, 0.3191) (-6.3262, 0.3371) knots 0 0 0 0 1 1 1 1
  spline S1391 degree 3 poles (-6.3262, 0.3371) (-5.8208, 0.3822) (-5.7486, 0.4364) (-6.1096, 0.5086) knots 0 0 0 0 1 1 1 1
  spline S1392 degree 3 poles (-6.1096, 0.5086) (-6.2811, 0.5447) (-6.4165, 0.644) (-6.4616, 0.7793) knots 0 0 0 0 1 1 1 1
  spline S1393 degree 3 poles (-6.4616, 0.7793) (-6.5248, 0.9508) (-6.615, 0.9959) (-6.8768, 1.005) knots 0 0 0 0 1 1 1 1
  spline S1394 degree 3 poles (-6.8768, 1.005) (-7.1385, 1.014) (-7.2017, 0.9869) (-7.1746, 0.8606) knots 0 0 0 0 1 1 1 1
  spline S1395 degree 3 poles (-7.1746, 0.8606) (-7.1565, 0.7703) (-7.0302, 0.6891) (-6.8768, 0.662) knots 0 0 0 0 1 1 1 1
  spline S1396 degree 3 poles (-6.8768, 0.662) (-6.5338, 0.5988) (-6.6241, 0.5447) (-7.4183, 0.3461) knots 0 0 0 0 1 1 1 1
  spline S1397 degree 3 poles (-7.4183, 0.3461) (-7.7702, 0.2559) (-8.0951, 0.1476) (-8.1403, 0.1025) knots 0 0 0 0 1 1 1 1
  spline S1398 degree 3 poles (-8.1403, 0.1025) (-8.1944, 0.0483) (-8.1764, 0.0393) (-8.0951, 0.0664) knots 0 0 0 0 1 1 1 1
  spline S1399 degree 3 poles (-8.0951, 0.0664) (-7.6258, 0.2108) (-7.4453, 0.2198) (-7.4905, 0.0844) knots 0 0 0 0 1 1 1 1
  spline S1400 degree 3 poles (-7.4905, 0.0844) (-7.5627, -0.0961) (-7.4905, -0.0961) (-7.0753, 0.1295) knots 0 0 0 0 1 1 1 1
  spline S1401 degree 3 poles (-9.0879, 0.2559) (-9.0157, 0.4635) (-9.0157, 0.6169) (-9.0789, 0.7252) knots 0 0 0 0 1 1 1 1
  spline S1402 degree 3 poles (-9.0789, 0.7252) (-9.1601, 0.8696) (-9.1781, 0.8606) (-9.2594, 0.6349) knots 0 0 0 0 1 1 1 1
  spline S1403 degree 3 poles (-9.2594, 0.6349) (-9.3767, 0.3191) (-9.3857, -0.06) (-9.2774, -0.06) knots 0 0 0 0 1 1 1 1
  spline S1404 degree 3 poles (-9.2774, -0.06) (-9.2323, -0.06) (-9.142, 0.0844) (-9.0879, 0.2559) knots 0 0 0 0 1 1 1 1
  spline S1405 degree 3 poles (-6.5609, 1.2938) (-6.5609, 1.3389) (-6.606, 1.384) (-6.6511, 1.384) knots 0 0 0 0 1 1 1 1
  spline S1406 degree 3 poles (-6.6511, 1.384) (-6.7053, 1.384) (-6.7414, 1.3389) (-6.7414, 1.2938) knots 0 0 0 0 1 1 1 1
  spline S1407 degree 3 poles (-6.7414, 1.2938) (-6.7414, 1.2396) (-6.7053, 1.2035) (-6.6511, 1.2035) knots 0 0 0 0 1 1 1 1
  spline S1408 degree 3 poles (-6.6511, 1.2035) (-6.606, 1.2035) (-6.5609, 1.2396) (-6.5609, 1.2938) knots 0 0 0 0 1 1 1 1
  spline S1409 degree 3 poles (-6.3804, 1.754) (-6.1548, 1.8533) (-5.9021, 1.9526) (-5.8118, 1.9887) knots 0 0 0 0 1 1 1 1
  spline S1410 degree 3 poles (-5.8118, 1.9887) (-5.6764, 2.0248) (-5.6674, 2.0609) (-5.7667, 2.115) knots 0 0 0 0 1 1 1 1
  spline S1411 degree 3 poles (-5.7667, 2.115) (-5.9291, 2.2233) (-6.2901, 2.2143) (-6.2901, 2.106) knots 0 0 0 0 1 1 1 1
  spline S1412 degree 3 poles (-6.2901, 2.106) (-6.2901, 2.0519) (-6.3443, 2.0158) (-6.4165, 2.0158) knots 0 0 0 0 1 1 1 1
  spline S1413 degree 3 poles (-6.4165, 2.0158) (-6.4797, 2.0158) (-6.606, 1.9165) (-6.6872, 1.7901) knots 0 0 0 0 1 1 1 1
  spline S1414 degree 3 poles (-6.6872, 1.7901) (-6.7685, 1.6638) (-6.8226, 1.5645) (-6.8136, 1.5735) knots 0 0 0 0 1 1 1 1
  spline S1415 degree 3 poles (-6.8136, 1.5735) (-6.7955, 1.5735) (-6.606, 1.6548) (-6.3804, 1.754) knots 0 0 0 0 1 1 1 1
  spline S1416 degree 3 poles (-9.1781, 2.0519) (-9.0608, 2.1692) (-9.0608, 2.3497) (-9.1781, 2.4219) knots 0 0 0 0 1 1 1 1
  spline S1417 degree 3 poles (-9.1781, 2.4219) (-9.2684, 2.476) (-9.6294, 2.1602) (-9.6294, 2.0248) knots 0 0 0 0 1 1 1 1
  spline S1418 degree 3 poles (-9.6294, 2.0248) (-9.6294, 1.9165) (-9.2955, 1.9345) (-9.1781, 2.0519) knots 0 0 0 0 1 1 1 1
  spline S1419 degree 3 poles (-10.4416, 2.097) (-10.4416, 2.1331) (-10.3333, 2.2865) (-10.207, 2.4309) knots 0 0 0 0 1 1 1 1
  spline S1420 degree 3 poles (-10.207, 2.4309) (-10.0626, 2.5753) (-10.0084, 2.7017) (-10.0716, 2.7197) knots 0 0 0 0 1 1 1 1
  spline S1421 degree 3 poles (-10.0716, 2.7197) (-10.1258, 2.7378) (-10.1709, 2.837) (-10.1709, 2.9453) knots 0 0 0 0 1 1 1 1
  spline S1422 degree 3 poles (-10.1709, 2.9453) (-10.1799, 3.1078) (-10.198, 3.0897) (-10.2972, 2.8641) knots 0 0 0 0 1 1 1 1
  spline S1423 degree 3 poles (-10.2972, 2.8641) (-10.3694, 2.7017) (-10.4868, 2.5392) (-10.559, 2.5031) knots 0 0 0 0 1 1 1 1
  spline S1424 degree 3 poles (-10.559, 2.5031) (-10.6312, 2.458) (-10.7214, 2.3316) (-10.7485, 2.2143) knots 0 0 0 0 1 1 1 1
  spline S1425 degree 3 poles (-10.7485, 2.2143) (-10.8026, 2.0519) (-10.7846, 2.0158) (-10.6312, 2.0158) knots 0 0 0 0 1 1 1 1
  spline S1426 degree 3 poles (-10.6312, 2.0158) (-10.5229, 2.0158) (-10.4416, 2.0519) (-10.4416, 2.097) knots 0 0 0 0 1 1 1 1
  spline S1427 degree 3 poles (-7.5085, 2.3768) (-7.4814, 2.4219) (-7.4995, 2.467) (-7.5446, 2.467) knots 0 0 0 0 1 1 1 1
  spline S1428 degree 3 poles (-7.5446, 2.467) (-7.5988, 2.467) (-7.6439, 2.4219) (-7.6439, 2.3768) knots 0 0 0 0 1 1 1 1
  spline S1429 degree 3 poles (-7.6439, 2.3768) (-7.6439, 2.3226) (-7.6258, 2.2865) (-7.6078, 2.2865) knots 0 0 0 0 1 1 1 1
  spline S1430 degree 3 poles (-7.6078, 2.2865) (-7.5807, 2.2865) (-7.5356, 2.3226) (-7.5085, 2.3768) knots 0 0 0 0 1 1 1 1
  spline S1431 degree 3 poles (-7.4183, 2.6475) (-7.671, 2.7558) (-8.0951, 2.7558) (-8.0951, 2.6475) knots 0 0 0 0 1 1 1 1
  spline S1432 degree 3 poles (-8.0951, 2.6475) (-8.0951, 2.5934) (-7.9056, 2.5573) (-7.671, 2.5663) knots 0 0 0 0 1 1 1 1
  spline S1433 degree 3 poles (-7.671, 2.5663) (-7.3461, 2.5663) (-7.2829, 2.5934) (-7.4183, 2.6475) knots 0 0 0 0 1 1 1 1
  spline S1434 degree 3 poles (-5.6584, 2.9995) (-5.6584, 3.0446) (-5.6313, 3.1439) (-5.6042, 3.2251) knots 0 0 0 0 1 1 1 1
  spline S1435 degree 3 poles (-5.6042, 3.2251) (-5.5681, 3.3334) (-5.6042, 3.3695) (-5.7396, 3.3695) knots 0 0 0 0 1 1 1 1
  spline S1436 degree 3 poles (-5.7396, 3.3695) (-5.9652, 3.3695) (-6.0104, 3.0536) (-5.7938, 2.9724) knots 0 0 0 0 1 1 1 1
  spline S1437 degree 3 poles (-5.7938, 2.9724) (-5.7216, 2.9453) (-5.6584, 2.9634) (-5.6584, 2.9995) knots 0 0 0 0 1 1 1 1
  spline S1438 degree 3 poles (-7.5988, 2.9995) (-7.5717, 3.0446) (-7.5807, 3.1078) (-7.6168, 3.1258) knots 0 0 0 0 1 1 1 1
  spline S1439 degree 3 poles (-7.6168, 3.1258) (-7.7341, 3.189) (-8.2756, 3.0897) (-8.2756, 2.9995) knots 0 0 0 0 1 1 1 1
  spline S1440 degree 3 poles (-8.2756, 2.9995) (-8.2756, 2.8912) (-7.671, 2.8912) (-7.5988, 2.9995) knots 0 0 0 0 1 1 1 1
  spline S1441 degree 3 poles (-10.6763, 3.0897) (-10.6402, 3.1349) (-10.6582, 3.198) (-10.7034, 3.2251) knots 0 0 0 0 1 1 1 1
  spline S1442 degree 3 poles (-10.7034, 3.2251) (-10.7485, 3.2612) (-10.8117, 3.2432) (-10.8387, 3.198) knots 0 0 0 0 1 1 1 1
  spline S1443 degree 3 poles (-10.8387, 3.198) (-10.8748, 3.1529) (-10.8568, 3.0897) (-10.8117, 3.0627) knots 0 0 0 0 1 1 1 1
  spline S1444 degree 3 poles (-10.8117, 3.0627) (-10.7665, 3.0266) (-10.7034, 3.0446) (-10.6763, 3.0897) knots 0 0 0 0 1 1 1 1
  spline S1445 degree 3 poles (-8.8171, 3.189) (-8.8171, 3.2341) (-8.8532, 3.2793) (-8.8984, 3.2793) knots 0 0 0 0 1 1 1 1
  spline S1446 degree 3 poles (-8.8984, 3.2793) (-8.9525, 3.2793) (-9.0157, 3.2341) (-9.0428, 3.189) knots 0 0 0 0 1 1 1 1
  spline S1447 degree 3 poles (-9.0428, 3.189) (-9.0698, 3.1349) (-9.0337, 3.0988) (-8.9615, 3.0988) knots 0 0 0 0 1 1 1 1
  spline S1448 degree 3 poles (-8.9615, 3.0988) (-8.8803, 3.0988) (-8.8171, 3.1349) (-8.8171, 3.189) knots 0 0 0 0 1 1 1 1
  spline S1449 degree 3 poles (14.35, -6.3955) (14.5486, -6.2963) (14.7471, -6.1248) (14.7832, -6.0255) knots 0 0 0 0 1 1 1 1
  spline S1450 degree 3 poles (14.7832, -6.0255) (14.8193, -5.9172) (15.045, -5.5291) (15.2977, -5.1501) knots 0 0 0 0 1 1 1 1
  spline S1451 degree 3 poles (15.2977, -5.1501) (16.0197, -4.0671) (15.9836, -3.4353) (15.1713, -3.2097) knots 0 0 0 0 1 1 1 1
  spline S1452 degree 3 poles (15.1713, -3.2097) (14.9547, -3.1465) (14.7381, -3.0653) (14.693, -3.0292) knots 0 0 0 0 1 1 1 1
  spline S1453 degree 3 poles (14.693, -3.0292) (14.6388, -2.9931) (14.2598, -2.966) (13.8356, -2.957) knots 0 0 0 0 1 1 1 1
  spline S1454 degree 3 poles (13.8356, -2.957) (13.4205, -2.948) (12.8338, -2.8848) (12.545, -2.8036) knots 0 0 0 0 1 1 1 1
  spline S1455 degree 3 poles (12.545, -2.8036) (12.0757, -2.6863) (11.9855, -2.6863) (11.7508, -2.8036) knots 0 0 0 0 1 1 1 1
  spline S1456 degree 3 poles (11.7508, -2.8036) (11.5974, -2.8758) (11.435, -2.9209) (11.3718, -2.9029) knots 0 0 0 0 1 1 1 1
  spline S1457 degree 3 poles (11.3718, -2.9029) (11.3086, -2.8758) (10.9205, -2.957) (10.4964, -3.0743) knots 0 0 0 0 1 1 1 1
  spline S1458 degree 3 poles (10.4964, -3.0743) (9.6029, -3.318) (9.4675, -3.4714) (9.5939, -4.0761) knots 0 0 0 0 1 1 1 1
  spline S1459 degree 3 poles (9.5939, -4.0761) (9.639, -4.2747) (9.7112, -4.6808) (9.7653, -4.9696) knots 0 0 0 0 1 1 1 1
  spline S1460 degree 3 poles (9.7653, -4.9696) (9.8195, -5.2674) (9.9639, -5.6555) (10.0812, -5.836) knots 0 0 0 0 1 1 1 1
  spline S1461 degree 3 poles (10.0812, -5.836) (10.4422, -6.3865) (10.74, -6.4677) (12.4548, -6.5219) knots 0 0 0 0 1 1 1 1
  spline S1462 degree 3 poles (12.4548, -6.5219) (13.8356, -6.567) (14.0071, -6.549) (14.35, -6.3955) knots 0 0 0 0 1 1 1 1
  spline S1463 degree 3 poles (10.4964, -5.6104) (10.3159, -5.4208) (10.2707, -5.2584) (10.2437, -4.771) knots 0 0 0 0 1 1 1 1
  spline S1464 degree 3 poles (10.2437, -4.771) (10.2166, -4.2476) (10.2346, -4.1303) (10.4151, -3.9046) knots 0 0 0 0 1 1 1 1
  spline S1465 degree 3 poles (10.4151, -3.9046) (10.7671, -3.4624) (11.0018, -3.4173) (12.888, -3.4624) knots 0 0 0 0 1 1 1 1
  spline S1466 degree 3 poles (12.888, -3.4624) (13.8266, -3.4805) (14.6298, -3.5256) (14.6659, -3.5617) knots 0 0 0 0 1 1 1 1
  spline S1467 degree 3 poles (14.6659, -3.5617) (14.7832, -3.679) (14.5035, -4.5635) (14.2869, -4.7981) knots 0 0 0 0 1 1 1 1
  spline S1468 degree 3 poles (14.2869, -4.7981) (14.1425, -4.9515) (13.7363, -5.132) (13.0685, -5.3396) knots 0 0 0 0 1 1 1 1
  spline S1469 degree 3 poles (13.0685, -5.3396) (11.2093, -5.9172) (10.8213, -5.9623) (10.4964, -5.6104) knots 0 0 0 0 1 1 1 1
  spline S1470 degree 3 poles (9.9097, -4.2115) (9.8827, -4.1664) (9.9007, -4.1212) (9.9458, -4.1212) knots 0 0 0 0 1 1 1 1
  spline S1471 degree 3 poles (9.9458, -4.1212) (10, -4.1212) (10.0451, -4.1664) (10.0451, -4.2115) knots 0 0 0 0 1 1 1 1
  spline S1472 degree 3 poles (10.0451, -4.2115) (10.0451, -4.2656) (10.0271, -4.3017) (10.009, -4.3017) knots 0 0 0 0 1 1 1 1
  spline S1473 degree 3 poles (10.009, -4.3017) (9.9819, -4.3017) (9.9368, -4.2656) (9.9097, -4.2115) knots 0 0 0 0 1 1 1 1
  spline S1474 degree 3 poles (16.0016, -2.8216) (16.0016, -2.7404) (15.9565, -2.6772) (15.9114, -2.6772) knots 0 0 0 0 1 1 1 1
  spline S1475 degree 3 poles (15.9114, -2.6772) (15.8572, -2.6772) (15.8211, -2.7133) (15.8211, -2.7585) knots 0 0 0 0 1 1 1 1
  spline S1476 degree 3 poles (15.8211, -2.7585) (15.8211, -2.8126) (15.8572, -2.8758) (15.9114, -2.9029) knots 0 0 0 0 1 1 1 1
  spline S1477 degree 3 poles (15.9114, -2.9029) (15.9565, -2.9299) (16.0016, -2.8938) (16.0016, -2.8216) knots 0 0 0 0 1 1 1 1
  spline S1478 degree 3 poles (15.2345, -2.5328) (15.6406, -2.4245) (15.776, -1.9101) (15.4691, -1.6033) knots 0 0 0 0 1 1 1 1
  spline S1479 degree 3 poles (15.4691, -1.6033) (15.2886, -1.4228) (14.8103, -1.3325) (13.7995, -1.2964) knots 0 0 0 0 1 1 1 1
  spline S1480 degree 3 poles (13.7995, -1.2964) (13.3212, -1.2784) (13.258, -1.3054) (13.0865, -1.522) knots 0 0 0 0 1 1 1 1
  line L82 (13.0865, -1.522) -> (12.906, -1.7567)
  line L83 (12.906, -1.7567) -> (13.1046, -2.0726)
  spline S1481 degree 3 poles (13.1046, -2.0726) (13.2129, -2.244) (13.3844, -2.4065) (13.5017, -2.4426) knots 0 0 0 0 1 1 1 1
  spline S1482 degree 3 poles (13.5017, -2.4426) (13.7995, -2.5238) (15.0269, -2.587) (15.2345, -2.5328) knots 0 0 0 0 1 1 1 1
  spline S1483 degree 3 poles (13.3573, -2.1448) (13.1046, -1.8921) (13.2129, -1.8108) (13.9168, -1.7386) knots 0 0 0 0 1 1 1 1
  spline S1484 degree 3 poles (13.9168, -1.7386) (14.5125, -1.6845) (15.1533, -1.7838) (15.3518, -1.9823) knots 0 0 0 0 1 1 1 1
  spline S1485 degree 3 poles (15.3518, -1.9823) (15.4691, -2.1087) (15.4691, -2.1448) (15.3608, -2.2801) knots 0 0 0 0 1 1 1 1
  spline S1486 degree 3 poles (15.3608, -2.2801) (15.2616, -2.4065) (15.1081, -2.4245) (14.3952, -2.3884) knots 0 0 0 0 1 1 1 1
  spline S1487 degree 3 poles (14.3952, -2.3884) (13.6822, -2.3433) (13.5197, -2.3072) (13.3573, -2.1448) knots 0 0 0 0 1 1 1 1
  spline S1488 degree 3 poles (15.0901, -2.235) (15.1713, -2.1809) (15.1803, -2.1357) (15.1081, -2.0996) knots 0 0 0 0 1 1 1 1
  spline S1489 degree 3 poles (15.1081, -2.0996) (14.9818, -2.0184) (14.6479, -2.1177) (14.6479, -2.235) knots 0 0 0 0 1 1 1 1
  spline S1490 degree 3 poles (14.6479, -2.235) (14.6479, -2.3343) (14.9186, -2.3433) (15.0901, -2.235) knots 0 0 0 0 1 1 1 1
  spline S1491 degree 3 poles (12.7707, -1.4679) (12.8338, -1.3506) (12.9782, -1.0979) (13.0775, -0.9083) knots 0 0 0 0 1 1 1 1
  spline S1492 degree 3 poles (13.0775, -0.9083) (13.3212, -0.4842) (13.61, -0.2044) (13.7363, -0.2856) knots 0 0 0 0 1 1 1 1
  spline S1493 degree 3 poles (13.7363, -0.2856) (13.7905, -0.3127) (13.8356, -0.3217) (13.8356, -0.2946) knots 0 0 0 0 1 1 1 1
  spline S1494 degree 3 poles (13.8356, -0.2946) (13.8356, -0.2676) (13.9078, -0.051) (13.9981, 0.1837) knots 0 0 0 0 1 1 1 1
  spline S1495 degree 3 poles (13.9981, 0.1837) (14.1425, 0.5537) (14.1515, 0.653) (14.0522, 0.8425) knots 0 0 0 0 1 1 1 1
  spline S1496 degree 3 poles (14.0522, 0.8425) (13.9259, 1.0772) (13.9349, 1.0952) (13.7544, 0.4183) knots 0 0 0 0 1 1 1 1
  spline S1497 degree 3 poles (13.7544, 0.4183) (13.6732, 0.1386) (13.5919, 0.0212) (13.4475, -0.0149) knots 0 0 0 0 1 1 1 1
  spline S1498 degree 3 poles (13.4475, -0.0149) (13.258, -0.069) (12.8429, -0.7549) (12.8429, -1.0166) knots 0 0 0 0 1 1 1 1
  spline S1499 degree 3 poles (12.8429, -1.0166) (12.8429, -1.0708) (12.7887, -1.1701) (12.7165, -1.2242) knots 0 0 0 0 1 1 1 1
  spline S1500 degree 3 poles (12.7165, -1.2242) (12.6443, -1.2874) (12.5902, -1.4137) (12.5992, -1.513) knots 0 0 0 0 1 1 1 1
  spline S1501 degree 3 poles (12.5992, -1.513) (12.6172, -1.7296) (12.6263, -1.7296) (12.7707, -1.4679) knots 0 0 0 0 1 1 1 1
  spline S1502 degree 3 poles (10.6137, -1.0979) (10.6588, -0.8) (10.7761, -0.4661) (10.8664, -0.3398) knots 0 0 0 0 1 1 1 1
  spline S1503 degree 3 poles (10.8664, -0.3398) (10.9927, -0.1863) (11.0379, 0.0212) (11.0379, 0.3822) knots 0 0 0 0 1 1 1 1
  spline S1504 degree 3 poles (11.0379, 0.3822) (11.0379, 0.6801) (11.0018, 0.8425) (10.9657, 0.7703) knots 0 0 0 0 1 1 1 1
  spline S1505 degree 3 poles (10.9657, 0.7703) (10.9205, 0.7071) (10.8303, 0.671) (10.7581, 0.6981) knots 0 0 0 0 1 1 1 1
  spline S1506 degree 3 poles (10.7581, 0.6981) (10.6859, 0.7162) (10.5234, 0.7613) (10.3881, 0.7884) knots 0 0 0 0 1 1 1 1
  spline S1507 degree 3 poles (10.3881, 0.7884) (10.0812, 0.8606) (9.8646, 1.2486) (9.8646, 1.745) knots 0 0 0 0 1 1 1 1
  spline S1508 degree 3 poles (9.8646, 1.745) (9.8646, 2.1692) (9.6841, 2.2324) (9.5397, 1.8533) knots 0 0 0 0 1 1 1 1
  spline S1509 degree 3 poles (9.5397, 1.8533) (9.4224, 1.5555) (9.4765, 1.2938) (9.6119, 1.4833) knots 0 0 0 0 1 1 1 1
  spline S1510 degree 3 poles (9.6119, 1.4833) (9.6751, 1.5826) (9.6841, 1.5645) (9.648, 1.4472) knots 0 0 0 0 1 1 1 1
  spline S1511 degree 3 poles (9.648, 1.4472) (9.6119, 1.3208) (9.7473, 1.0952) (10.1354, 0.644) knots 0 0 0 0 1 1 1 1
  spline S1512 degree 3 poles (10.1354, 0.644) (10.4332, 0.301) (10.6769, -0.0149) (10.6769, -0.051) knots 0 0 0 0 1 1 1 1
  spline S1513 degree 3 poles (10.6769, -0.051) (10.6769, -0.0871) (10.6317, -0.2495) (10.5776, -0.3939) knots 0 0 0 0 1 1 1 1
  spline S1514 degree 3 poles (10.5776, -0.3939) (10.5325, -0.5473) (10.4964, -0.8903) (10.5144, -1.152) knots 0 0 0 0 1 1 1 1
  line L84 (10.5144, -1.152) -> (10.5415, -1.6394)
  line L85 (10.5415, -1.6394) -> (10.6137, -1.0979)
  spline S1515 degree 3 poles (10.2256, -1.513) (10.2256, -1.4589) (10.1805, -1.3957) (10.1354, -1.3686) knots 0 0 0 0 1 1 1 1
  spline S1516 degree 3 poles (10.1354, -1.3686) (10.0812, -1.3415) (10.0451, -1.3776) (10.0451, -1.4498) knots 0 0 0 0 1 1 1 1
  spline S1517 degree 3 poles (10.0451, -1.4498) (10.0451, -1.5311) (10.0812, -1.5942) (10.1354, -1.5942) knots 0 0 0 0 1 1 1 1
  spline S1518 degree 3 poles (10.1354, -1.5942) (10.1805, -1.5942) (10.2256, -1.5581) (10.2256, -1.513) knots 0 0 0 0 1 1 1 1
  spline S1519 degree 3 poles (11.1642, -1.4408) (11.2635, -1.3325) (11.2184, -0.9896) (11.083, -0.8722) knots 0 0 0 0 1 1 1 1
  spline S1520 degree 3 poles (11.083, -0.8722) (10.9657, -0.773) (10.9476, -0.8091) (10.9476, -1.0798) knots 0 0 0 0 1 1 1 1
  spline S1521 degree 3 poles (10.9476, -1.0798) (10.9476, -1.3957) (11.0469, -1.5581) (11.1642, -1.4408) knots 0 0 0 0 1 1 1 1
  spline S1522 degree 3 poles (11.5794, -1.3325) (11.5794, -1.2784) (11.5433, -1.2152) (11.4891, -1.1881) knots 0 0 0 0 1 1 1 1
  spline S1523 degree 3 poles (11.4891, -1.1881) (11.435, -1.161) (11.4259, -1.1971) (11.453, -1.2693) knots 0 0 0 0 1 1 1 1
  spline S1524 degree 3 poles (11.453, -1.2693) (11.5162, -1.4318) (11.5794, -1.4589) (11.5794, -1.3325) knots 0 0 0 0 1 1 1 1
  spline S1525 degree 3 poles (10.2527, -0.5203) (10.3159, -0.1141) (10.2978, -0.0239) (10.1624, 0.0844) knots 0 0 0 0 1 1 1 1
  spline S1526 degree 3 poles (10.1624, 0.0844) (10, 0.2108) (9.8466, 0.2108) (9.8556, 0.0934) knots 0 0 0 0 1 1 1 1
  spline S1527 degree 3 poles (9.8556, 0.0934) (9.8646, 0.0573) (9.8646, -0.051) (9.8646, -0.1502) knots 0 0 0 0 1 1 1 1
  spline S1528 degree 3 poles (9.8646, -0.1502) (9.8646, -0.2495) (9.9188, -0.3307) (9.991, -0.3307) knots 0 0 0 0 1 1 1 1
  spline S1529 degree 3 poles (9.991, -0.3307) (10.0812, -0.3307) (10.1354, -0.4481) (10.1534, -0.6737) knots 0 0 0 0 1 1 1 1
  spline S1530 degree 3 poles (10.1534, -0.6737) (10.1805, -0.9896) (10.1805, -0.9805) (10.2527, -0.5203) knots 0 0 0 0 1 1 1 1
  spline S1531 degree 3 poles (14.0432, -0.6917) (13.9259, -0.5744) (13.8085, -0.5293) (13.7093, -0.5654) knots 0 0 0 0 1 1 1 1
  spline S1532 degree 3 poles (13.7093, -0.5654) (13.4746, -0.6556) (13.5919, -0.8271) (13.9168, -0.8542) knots 0 0 0 0 1 1 1 1
  line L86 (13.9168, -0.8542) -> (14.2147, -0.8813)
  line L87 (14.2147, -0.8813) -> (14.0432, -0.6917)
  spline S1533 degree 3 poles (12.6985, -0.7369) (12.7346, -0.6376) (12.7977, -0.4932) (12.8429, -0.4029) knots 0 0 0 0 1 1 1 1
  spline S1534 degree 3 poles (12.8429, -0.4029) (12.897, -0.3037) (12.888, -0.2405) (12.7887, -0.2044) knots 0 0 0 0 1 1 1 1
  spline S1535 degree 3 poles (12.7887, -0.2044) (12.6263, -0.1412) (12.545, -0.3217) (12.5902, -0.6647) knots 0 0 0 0 1 1 1 1
  spline S1536 degree 3 poles (12.5902, -0.6647) (12.6263, -0.8903) (12.6353, -0.8993) (12.6985, -0.7369) knots 0 0 0 0 1 1 1 1
  spline S1537 degree 3 poles (14.3591, -0.1322) (14.5305, 0.0393) (14.4854, 0.1386) (14.2598, 0.1025) knots 0 0 0 0 1 1 1 1
  spline S1538 degree 3 poles (14.2598, 0.1025) (14.1515, 0.0844) (14.0612, 0.0212) (14.0612, -0.051) knots 0 0 0 0 1 1 1 1
  spline S1539 degree 3 poles (14.0612, -0.051) (14.0612, -0.2224) (14.2237, -0.2676) (14.3591, -0.1322) knots 0 0 0 0 1 1 1 1
  spline S1540 degree 3 poles (11.7869, 0.2559) (11.823, 0.3281) (11.805, 0.4093) (11.7599, 0.4364) knots 0 0 0 0 1 1 1 1
  spline S1541 degree 3 poles (11.7599, 0.4364) (11.7057, 0.4725) (11.6696, 0.4725) (11.6696, 0.4454) knots 0 0 0 0 1 1 1 1
  spline S1542 degree 3 poles (11.6696, 0.4454) (11.6696, 0.4274) (11.6425, 0.3461) (11.6155, 0.2649) knots 0 0 0 0 1 1 1 1
  spline S1543 degree 3 poles (11.6155, 0.2649) (11.5884, 0.1837) (11.5974, 0.1205) (11.6516, 0.1205) knots 0 0 0 0 1 1 1 1
  spline S1544 degree 3 poles (11.6516, 0.1205) (11.6967, 0.1205) (11.7599, 0.1837) (11.7869, 0.2559) knots 0 0 0 0 1 1 1 1
  spline S1545 degree 3 poles (11.3989, 0.4093) (11.3989, 0.5266) (11.462, 0.7342) (11.5342, 0.8696) knots 0 0 0 0 1 1 1 1
  spline S1546 degree 3 poles (11.5342, 0.8696) (11.6606, 1.1223) (11.6245, 1.6909) (11.4801, 1.6096) knots 0 0 0 0 1 1 1 1
  spline S1547 degree 3 poles (11.4801, 1.6096) (11.444, 1.5826) (11.3808, 1.366) (11.3537, 1.1313) knots 0 0 0 0 1 1 1 1
  spline S1548 degree 3 poles (11.3537, 1.1313) (11.3267, 0.8967) (11.2815, 0.5988) (11.2635, 0.4544) knots 0 0 0 0 1 1 1 1
  spline S1549 degree 3 poles (11.2635, 0.4544) (11.2364, 0.3191) (11.2635, 0.2108) (11.3086, 0.2108) knots 0 0 0 0 1 1 1 1
  spline S1550 degree 3 poles (11.3086, 0.2108) (11.3628, 0.2108) (11.3989, 0.301) (11.3989, 0.4093) knots 0 0 0 0 1 1 1 1
  spline S1551 degree 3 poles (13.5649, 1.3389) (13.5649, 1.8082) (13.5378, 2.1963) (13.5107, 2.1963) knots 0 0 0 0 1 1 1 1
  spline S1552 degree 3 poles (13.5107, 2.1963) (13.4746, 2.1963) (13.3753, 2.115) (13.2851, 2.0067) knots 0 0 0 0 1 1 1 1
  spline S1553 degree 3 poles (13.2851, 2.0067) (13.1317, 1.8353) (13.1226, 1.8353) (13.0234, 1.9887) knots 0 0 0 0 1 1 1 1
  spline S1554 degree 3 poles (13.0234, 1.9887) (12.9421, 2.1241) (12.9331, 2.106) (12.9782, 1.8894) knots 0 0 0 0 1 1 1 1